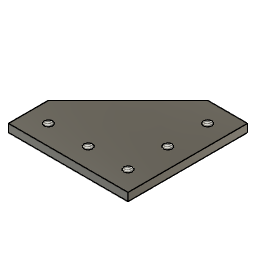
bracket_plate (Autodesk Fusion 360 design; units mm, degrees)
Autodesk Fusion 360 part; units mm, degrees
sketch "Sketch1" plane through (0, 0, 0) normal (0, 0, 1) x (1, 0, 0)
  line L0 (0, 0) -> (60, 0)
  line L1 (60, 0) -> (60, 60)
  line L2 (60, 60) -> (40, 60)
  line L3 (0, 0) -> (0, 20)
  line L4 (0, 20) -> (40, 60)
  dimension "d1" = 60
  dimension "d2" = 60
  dimension "d3" = 20
  dimension "d4" = 20
  constraint coincident L0.start L3.start
  constraint horizontal L0
  constraint perpendicular L0 L1
  constraint perpendicular L1 L2
  constraint perpendicular L2 L3
  measures "d1" distance of L0.start L0.end
  measures "d2" distance of L0.end L1.end
  measures "d3" distance of L1.end L2.end
  measures "d4" distance of L0.start L3.end
extrude "Extrude1" add sketch "Sketch1" along normal blind 4
hole "Hole2" at (10, 10, 4) direction (0, 0, -1) diameter 4.234 depth 34 tip angle 180
thread "Thread2" "ANSI Metric M Profile 5.0 M5x0.8 6H" thread offset 0 thread depth 7.4
hole "Hole3" at (50, 10, 4) direction (0, 0, -1) diameter 4.234 depth 34 tip angle 180
thread "Thread3" "ANSI Metric M Profile 5.0 M5x0.8 6H" thread offset 0 thread depth 7.4
hole "Hole4" at (50, 50, 4) direction (0, 0, -1) diameter 4.234 depth 34 tip angle 180
thread "Thread4" "ANSI Metric M Profile 5.0 M5x0.8 6H" thread offset 0 thread depth 7.4
hole "Hole5" at (50, 30, 4) direction (0, 0, -1) diameter 4.234 depth 34 tip angle 180
thread "Thread5" "ANSI Metric M Profile 5.0 M5x0.8 6H" thread offset 0 thread depth 7.4
hole "Hole6" at (30, 10, 4) direction (0, 0, -1) diameter 4.234 depth 34 tip angle 180
thread "Thread6" "ANSI Metric M Profile 5.0 M5x0.8 6H" thread offset 0 thread depth 7.4
